Autodesk Fusion 360 part; units mm, degrees
(part 2 of 9)
sketch "Sketch3" plane through (0, 0, 5) normal (0, 0, 1) x (-1, 0, 0)
  line L0 (-9.15, 99.3) -> (-24.15, 99.3)
  line L1 (-24.15, 99.3) -> (-24.15, 114.3)
  line L2 (-24.15, 114.3) -> (-9.15, 114.3)
  line L3 (-9.15, 114.3) -> (-9.15, 99.3)
  line L4 (-42.475, 99.3) -> (-57.475, 99.3)
  line L5 (-57.475, 99.3) -> (-57.475, 114.3)
  line L6 (-57.475, 114.3) -> (-42.475, 114.3)
  line L7 (-42.475, 114.3) -> (-42.475, 99.3)
  line L8 (42.5, 114.3) -> (57.5, 114.3)
  line L9 (57.5, 114.3) -> (57.5, 99.3)
  line L10 (57.5, 99.3) -> (42.5, 99.3)
  line L11 (42.5, 99.3) -> (42.5, 114.3)
  line L12 (24.175, 99.3) -> (9.175, 99.3)
  line L13 (9.175, 99.3) -> (9.175, 114.3)
  line L14 (9.175, 114.3) -> (24.175, 114.3)
  line L15 (24.175, 114.3) -> (24.175, 99.3)
  line L16 (-76.5, 75.505) -> (-91.5, 75.505)
  line L17 (-91.5, 75.505) -> (-91.5, 90.505)
  line L18 (-91.5, 90.505) -> (-76.5, 90.505)
  line L19 (-76.5, 90.505) -> (-76.5, 75.505)
  line L20 (-59.7, 75.505) -> (-74.7, 75.505)
  line L21 (-74.7, 75.505) -> (-74.7, 90.505)
  line L22 (-74.7, 90.505) -> (-59.7, 90.505)
  line L23 (-59.7, 90.505) -> (-59.7, 75.505)
  line L24 (-42.9, 75.505) -> (-57.9, 75.505)
  line L25 (-57.9, 75.505) -> (-57.9, 90.505)
  line L26 (-57.9, 90.505) -> (-42.9, 90.505)
  line L27 (-42.9, 90.505) -> (-42.9, 75.505)
  line L28 (-9.3, -72.055) -> (-24.3, -72.055)
  line L29 (-24.3, -72.055) -> (-24.3, -57.055)
  line L30 (-24.3, -57.055) -> (-9.3, -57.055)
  line L31 (-9.3, -57.055) -> (-9.3, -72.055)
  line L32 (24.3, -72.055) -> (9.3, -72.055)
  line L33 (9.3, -72.055) -> (9.3, -57.055)
  line L34 (9.3, -57.055) -> (24.3, -57.055)
  line L35 (24.3, -57.055) -> (24.3, -72.055)
  line L36 (57.9, -72.055) -> (42.9, -72.055)
  line L37 (42.9, -72.055) -> (42.9, -57.055)
  line L38 (42.9, -57.055) -> (57.9, -57.055)
  line L39 (57.9, -57.055) -> (57.9, -72.055)
  line L40 (41.1, -72.055) -> (26.1, -72.055)
  line L41 (26.1, -72.055) -> (26.1, -57.055)
  line L42 (26.1, -57.055) -> (41.1, -57.055)
  line L43 (41.1, -57.055) -> (41.1, -72.055)
  line L44 (-76.5, -90.5) -> (-91.5, -90.5)
  line L45 (-91.5, -90.5) -> (-91.5, -75.5)
  line L46 (-91.5, -75.5) -> (-76.5, -75.5)
  line L47 (-76.5, -75.5) -> (-76.5, -90.5)
  line L48 (91.5, -72.055) -> (76.5, -72.055)
  line L49 (76.5, -72.055) -> (76.5, -57.055)
  line L50 (76.5, -57.055) -> (91.5, -57.055)
  line L51 (91.5, -57.055) -> (91.5, -72.055)
  line L52 (7.5, -72.055) -> (-7.5, -72.055)
  line L53 (-7.5, -72.055) -> (-7.5, -57.055)
  line L54 (-7.5, -57.055) -> (7.5, -57.055)
  line L55 (7.5, -57.055) -> (7.5, -72.055)
  line L56 (74.7, -72.055) -> (59.7, -72.055)
  line L57 (59.7, -72.055) -> (59.7, -57.055)
  line L58 (59.7, -57.055) -> (74.7, -57.055)
  line L59 (74.7, -57.055) -> (74.7, -72.055)
  line L60 (24.3, -90.5) -> (9.3, -90.5)
  line L61 (9.3, -90.5) -> (9.3, -75.5)
  line L62 (9.3, -75.5) -> (24.3, -75.5)
  line L63 (24.3, -75.5) -> (24.3, -90.5)
  line L64 (7.5, -90.5) -> (-7.5, -90.5)
  line L65 (-7.5, -90.5) -> (-7.5, -75.5)
  line L66 (-7.5, -75.5) -> (7.5, -75.5)
  line L67 (7.5, -75.5) -> (7.5, -90.5)
  line L68 (-59.7, -90.5) -> (-74.7, -90.5)
  line L69 (-74.7, -90.5) -> (-74.7, -75.5)
  line L70 (-74.7, -75.5) -> (-59.7, -75.5)
  line L71 (-59.7, -75.5) -> (-59.7, -90.5)
  line L72 (-9.3, -90.5) -> (-24.3, -90.5)
  line L73 (-24.3, -90.5) -> (-24.3, -75.5)
  line L74 (-24.3, -75.5) -> (-9.3, -75.5)
  line L75 (-9.3, -75.5) -> (-9.3, -90.5)
  line L76 (41.1, -90.5) -> (26.1, -90.5)
  line L77 (26.1, -90.5) -> (26.1, -75.5)
  line L78 (26.1, -75.5) -> (41.1, -75.5)
  line L79 (41.1, -75.5) -> (41.1, -90.5)
  line L80 (-26.1, -90.5) -> (-41.1, -90.5)
  line L81 (-41.1, -90.5) -> (-41.1, -75.5)
  line L82 (-41.1, -75.5) -> (-26.1, -75.5)
  line L83 (-26.1, -75.5) -> (-26.1, -90.5)
  line L84 (-42.9, -90.5) -> (-57.9, -90.5)
  line L85 (-57.9, -90.5) -> (-57.9, -75.5)
  line L86 (-57.9, -75.5) -> (-42.9, -75.5)
  line L87 (-42.9, -75.5) -> (-42.9, -90.5)
  circle A0 centre (110, 110) radius 1.6
  line L88 (76.5, -75.5) -> (91.5, -75.5)
  line L89 (91.5, -75.5) -> (91.5, -90.5)
  line L90 (91.5, -90.5) -> (76.5, -90.5)
  line L91 (76.5, -90.5) -> (76.5, -75.5)
  line L92 (74.7, -90.5) -> (59.7, -90.5)
  line L93 (59.7, -90.5) -> (59.7, -75.5)
  line L94 (59.7, -75.5) -> (74.7, -75.5)
  line L95 (74.7, -75.5) -> (74.7, -90.5)
  line L96 (57.9, -90.5) -> (42.9, -90.5)
  line L97 (42.9, -90.5) -> (42.9, -75.5)
  line L98 (42.9, -75.5) -> (57.9, -75.5)
  line L99 (57.9, -75.5) -> (57.9, -90.5)
  circle A1 centre (-110, -110) radius 1.6
  circle A2 centre (-110, 110) radius 1.6
  line L100 (-76.5, -72.055) -> (-91.5, -72.055)
  line L101 (-91.5, -72.055) -> (-91.5, -57.055)
  line L102 (-91.5, -57.055) -> (-76.5, -57.055)
  line L103 (-76.5, -57.055) -> (-76.5, -72.055)
  line L104 (91.5, -53.61) -> (76.5, -53.61)
  line L105 (76.5, -53.61) -> (76.5, -38.61)
  line L106 (76.5, -38.61) -> (91.5, -38.61)
  line L107 (91.5, -38.61) -> (91.5, -53.61)
  circle A3 centre (110, -110) radius 1.6
  line L108 (-42.9, -72.055) -> (-57.9, -72.055)
  line L109 (-57.9, -72.055) -> (-57.9, -57.055)
  line L110 (-57.9, -57.055) -> (-42.9, -57.055)
  line L111 (-42.9, -57.055) -> (-42.9, -72.055)
  line L112 (-26.1, -72.055) -> (-41.1, -72.055)
  line L113 (-41.1, -72.055) -> (-41.1, -57.055)
  line L114 (-41.1, -57.055) -> (-26.1, -57.055)
  line L115 (-26.1, -57.055) -> (-26.1, -72.055)
  line L116 (-59.7, -72.055) -> (-74.7, -72.055)
  line L117 (-74.7, -72.055) -> (-74.7, -57.055)
  line L118 (-74.7, -57.055) -> (-59.7, -57.055)
  line L119 (-59.7, -57.055) -> (-59.7, -72.055)
  line L120 (74.7, -53.61) -> (59.7, -53.61)
  line L121 (59.7, -53.61) -> (59.7, -38.61)
  line L122 (59.7, -38.61) -> (74.7, -38.61)
  line L123 (74.7, -38.61) -> (74.7, -53.61)
  line L124 (57.9, -53.61) -> (42.9, -53.61)
  line L125 (42.9, -53.61) -> (42.9, -38.61)
  line L126 (42.9, -38.61) -> (57.9, -38.61)
  line L127 (57.9, -38.61) -> (57.9, -53.61)
  line L128 (41.1, -35.165) -> (26.1, -35.165)
  line L129 (26.1, -35.165) -> (26.1, -20.165)
  line L130 (26.1, -20.165) -> (41.1, -20.165)
  line L131 (41.1, -20.165) -> (41.1, -35.165)
  line L132 (24.3, -35.165) -> (9.3, -35.165)
  line L133 (9.3, -35.165) -> (9.3, -20.165)
  line L134 (9.3, -20.165) -> (24.3, -20.165)
  line L135 (24.3, -20.165) -> (24.3, -35.165)
  line L136 (7.5, -35.165) -> (-7.5, -35.165)
  line L137 (-7.5, -35.165) -> (-7.5, -20.165)
  line L138 (-7.5, -20.165) -> (7.5, -20.165)
  line L139 (7.5, -20.165) -> (7.5, -35.165)
  line L140 (-26.1, -35.165) -> (-41.1, -35.165)
  line L141 (-41.1, -35.165) -> (-41.1, -20.165)
  line L142 (-41.1, -20.165) -> (-26.1, -20.165)
  line L143 (-26.1, -20.165) -> (-26.1, -35.165)
  line L144 (-9.3, -35.165) -> (-24.3, -35.165)
  line L145 (-24.3, -35.165) -> (-24.3, -20.165)
  line L146 (-24.3, -20.165) -> (-9.3, -20.165)
  line L147 (-9.3, -20.165) -> (-9.3, -35.165)
  line L148 (-42.9, -35.165) -> (-57.9, -35.165)
  line L149 (-57.9, -35.165) -> (-57.9, -20.165)
  line L150 (-57.9, -20.165) -> (-42.9, -20.165)
  line L151 (-42.9, -20.165) -> (-42.9, -35.165)
  line L152 (-59.7, -35.165) -> (-74.7, -35.165)
  line L153 (-74.7, -35.165) -> (-74.7, -20.165)
  line L154 (-74.7, -20.165) -> (-59.7, -20.165)
  line L155 (-59.7, -20.165) -> (-59.7, -35.165)
  line L156 (41.1, -16.72) -> (26.1, -16.72)
  line L157 (26.1, -16.72) -> (26.1, -1.72)
  line L158 (26.1, -1.72) -> (41.1, -1.72)
  line L159 (41.1, -1.72) -> (41.1, -16.72)
  line L160 (91.5, -16.72) -> (76.5, -16.72)
  line L161 (76.5, -16.72) -> (76.5, -1.72)
  line L162 (76.5, -1.72) -> (91.5, -1.72)
  line L163 (91.5, -1.72) -> (91.5, -16.72)
  line L164 (74.7, -16.72) -> (59.7, -16.72)
  line L165 (59.7, -16.72) -> (59.7, -1.72)
  line L166 (59.7, -1.72) -> (74.7, -1.72)
  line L167 (74.7, -1.72) -> (74.7, -16.72)
  line L168 (57.9, -16.72) -> (42.9, -16.72)
  line L169 (42.9, -16.72) -> (42.9, -1.72)
  line L170 (42.9, -1.72) -> (57.9, -1.72)
  line L171 (57.9, -1.72) -> (57.9, -16.72)
  line L172 (24.3, -16.72) -> (9.3, -16.72)
  line L173 (9.3, -16.72) -> (9.3, -1.72)
  line L174 (9.3, -1.72) -> (24.3, -1.72)
  line L175 (24.3, -1.72) -> (24.3, -16.72)
  line L176 (7.5, -16.72) -> (-7.5, -16.72)
  line L177 (-7.5, -16.72) -> (-7.5, -1.72)
  line L178 (-7.5, -1.72) -> (7.5, -1.72)
  line L179 (7.5, -1.72) -> (7.5, -16.72)
  line L180 (-76.5, -35.165) -> (-91.5, -35.165)
  line L181 (-91.5, -35.165) -> (-91.5, -20.165)
  line L182 (-91.5, -20.165) -> (-76.5, -20.165)
  line L183 (-76.5, -20.165) -> (-76.5, -35.165)
  line L184 (-42.9, -16.72) -> (-57.9, -16.72)
  line L185 (-57.9, -16.72) -> (-57.9, -1.72)
  line L186 (-57.9, -1.72) -> (-42.9, -1.72)
  line L187 (-42.9, -1.72) -> (-42.9, -16.72)
  line L188 (-59.7, -16.72) -> (-74.7, -16.72)
  line L189 (-74.7, -16.72) -> (-74.7, -1.72)
  line L190 (-74.7, -1.72) -> (-59.7, -1.72)
  line L191 (-59.7, -1.72) -> (-59.7, -16.72)
  line L192 (-9.3, -16.72) -> (-24.3, -16.72)
  line L193 (-24.3, -16.72) -> (-24.3, -1.72)
  line L194 (-24.3, -1.72) -> (-9.3, -1.72)
  line L195 (-9.3, -1.72) -> (-9.3, -16.72)
  line L196 (-26.1, -16.72) -> (-41.1, -16.72)
  line L197 (-41.1, -16.72) -> (-41.1, -1.72)
  line L198 (-41.1, -1.72) -> (-26.1, -1.72)
  line L199 (-26.1, -1.72) -> (-26.1, -16.72)
  line L200 (-9.3, -53.61) -> (-24.3, -53.61)
  line L201 (-24.3, -53.61) -> (-24.3, -38.61)
  line L202 (-24.3, -38.61) -> (-9.3, -38.61)
  line L203 (-9.3, -38.61) -> (-9.3, -53.61)
  line L204 (7.5, -53.61) -> (-7.5, -53.61)
  line L205 (-7.5, -53.61) -> (-7.5, -38.61)
  line L206 (-7.5, -38.61) -> (7.5, -38.61)
  line L207 (7.5, -38.61) -> (7.5, -53.61)
  line L208 (24.3, -53.61) -> (9.3, -53.61)
  line L209 (9.3, -53.61) -> (9.3, -38.61)
  line L210 (9.3, -38.61) -> (24.3, -38.61)
  line L211 (24.3, -38.61) -> (24.3, -53.61)
  line L212 (41.1, -53.61) -> (26.1, -53.61)
  line L213 (26.1, -53.61) -> (26.1, -38.61)
  line L214 (26.1, -38.61) -> (41.1, -38.61)
  line L215 (41.1, -38.61) -> (41.1, -53.61)
  line L216 (91.5, -35.165) -> (76.5, -35.165)
  line L217 (76.5, -35.165) -> (76.5, -20.165)
  line L218 (76.5, -20.165) -> (91.5, -20.165)
  line L219 (91.5, -20.165) -> (91.5, -35.165)
  line L220 (57.9, -35.165) -> (42.9, -35.165)
  line L221 (42.9, -35.165) -> (42.9, -20.165)
  line L222 (42.9, -20.165) -> (57.9, -20.165)
  line L223 (57.9, -20.165) -> (57.9, -35.165)
  line L224 (-76.5, -53.61) -> (-91.5, -53.61)
  line L225 (-91.5, -53.61) -> (-91.5, -38.61)
  line L226 (-91.5, -38.61) -> (-76.5, -38.61)
  line L227 (-76.5, -38.61) -> (-76.5, -53.61)
  line L228 (-59.7, -53.61) -> (-74.7, -53.61)
  line L229 (-74.7, -53.61) -> (-74.7, -38.61)
  line L230 (-74.7, -38.61) -> (-59.7, -38.61)
  line L231 (-59.7, -38.61) -> (-59.7, -53.61)
  line L232 (-26.1, -53.61) -> (-41.1, -53.61)
  line L233 (-41.1, -53.61) -> (-41.1, -38.61)
  line L234 (-41.1, -38.61) -> (-26.1, -38.61)
  line L235 (-26.1, -38.61) -> (-26.1, -53.61)
  line L236 (74.7, -35.165) -> (59.7, -35.165)
  line L237 (59.7, -35.165) -> (59.7, -20.165)
  line L238 (59.7, -20.165) -> (74.7, -20.165)
  line L239 (74.7, -20.165) -> (74.7, -35.165)
  line L240 (-42.9, -53.61) -> (-57.9, -53.61)
  line L241 (-57.9, -53.61) -> (-57.9, -38.61)
  line L242 (-57.9, -38.61) -> (-42.9, -38.61)
  line L243 (-42.9, -38.61) -> (-42.9, -53.61)
  line L244 (41.1, 38.615) -> (26.1, 38.615)
  line L245 (26.1, 38.615) -> (26.1, 53.615)
  line L246 (26.1, 53.615) -> (41.1, 53.615)
  line L247 (41.1, 53.615) -> (41.1, 38.615)
  line L248 (91.5, 38.615) -> (76.5, 38.615)
  line L249 (76.5, 38.615) -> (76.5, 53.615)
  line L250 (76.5, 53.615) -> (91.5, 53.615)
  line L251 (91.5, 53.615) -> (91.5, 38.615)
  line L252 (7.5, 38.615) -> (-7.5, 38.615)
  line L253 (-7.5, 38.615) -> (-7.5, 53.615)
  line L254 (-7.5, 53.615) -> (7.5, 53.615)
  line L255 (7.5, 53.615) -> (7.5, 38.615)
  line L256 (74.7, 38.615) -> (59.7, 38.615)
  line L257 (59.7, 38.615) -> (59.7, 53.615)
  line L258 (59.7, 53.615) -> (74.7, 53.615)
  line L259 (74.7, 53.615) -> (74.7, 38.615)
  line L260 (24.3, 38.615) -> (9.3, 38.615)
  line L261 (9.3, 38.615) -> (9.3, 53.615)
  line L262 (9.3, 53.615) -> (24.3, 53.615)
  line L263 (24.3, 53.615) -> (24.3, 38.615)
  line L264 (57.9, 38.615) -> (42.9, 38.615)
  line L265 (42.9, 38.615) -> (42.9, 53.615)
  line L266 (42.9, 53.615) -> (57.9, 53.615)
  line L267 (57.9, 53.615) -> (57.9, 38.615)
  line L268 (91.5, 57.06) -> (76.5, 57.06)
  line L269 (76.5, 57.06) -> (76.5, 72.06)
  line L270 (76.5, 72.06) -> (91.5, 72.06)
  line L271 (91.5, 72.06) -> (91.5, 57.06)
  line L272 (-59.7, 38.615) -> (-74.7, 38.615)
  line L273 (-74.7, 38.615) -> (-74.7, 53.615)
  line L274 (-74.7, 53.615) -> (-59.7, 53.615)
  line L275 (-59.7, 53.615) -> (-59.7, 38.615)
  line L276 (-42.9, 38.615) -> (-57.9, 38.615)
  line L277 (-57.9, 38.615) -> (-57.9, 53.615)
  line L278 (-57.9, 53.615) -> (-42.9, 53.615)
  line L279 (-42.9, 53.615) -> (-42.9, 38.615)
  line L280 (-26.1, 38.615) -> (-41.1, 38.615)
  line L281 (-41.1, 38.615) -> (-41.1, 53.615)
  line L282 (-41.1, 53.615) -> (-26.1, 53.615)
  line L283 (-26.1, 53.615) -> (-26.1, 38.615)
  line L284 (-76.5, 38.615) -> (-91.5, 38.615)
  line L285 (-91.5, 38.615) -> (-91.5, 53.615)
  line L286 (-91.5, 53.615) -> (-76.5, 53.615)
  line L287 (-76.5, 53.615) -> (-76.5, 38.615)
  line L288 (-9.3, 38.615) -> (-24.3, 38.615)
  line L289 (-24.3, 38.615) -> (-24.3, 53.615)
  line L290 (-24.3, 53.615) -> (-9.3, 53.615)
  line L291 (-9.3, 53.615) -> (-9.3, 38.615)
  line L292 (57.9, 57.06) -> (42.9, 57.06)
  line L293 (42.9, 57.06) -> (42.9, 72.06)
  line L294 (42.9, 72.06) -> (57.9, 72.06)
  line L295 (57.9, 72.06) -> (57.9, 57.06)
  line L296 (24.3, 57.06) -> (9.3, 57.06)
  line L297 (9.3, 57.06) -> (9.3, 72.06)
  line L298 (9.3, 72.06) -> (24.3, 72.06)
  line L299 (24.3, 72.06) -> (24.3, 57.06)
  line L300 (41.1, 57.06) -> (26.1, 57.06)
  line L301 (26.1, 57.06) -> (26.1, 72.06)
  line L302 (26.1, 72.06) -> (41.1, 72.06)
  line L303 (41.1, 72.06) -> (41.1, 57.06)
  line L304 (-9.3, 57.06) -> (-24.3, 57.06)
  line L305 (-24.3, 57.06) -> (-24.3, 72.06)
  line L306 (-24.3, 72.06) -> (-9.3, 72.06)
  line L307 (-9.3, 72.06) -> (-9.3, 57.06)
  line L308 (7.5, 57.06) -> (-7.5, 57.06)
  line L309 (-7.5, 57.06) -> (-7.5, 72.06)
  line L310 (-7.5, 72.06) -> (7.5, 72.06)
  line L311 (7.5, 72.06) -> (7.5, 57.06)
  line L312 (74.7, 57.06) -> (59.7, 57.06)
  line L313 (59.7, 57.06) -> (59.7, 72.06)
  line L314 (59.7, 72.06) -> (74.7, 72.06)
  line L315 (74.7, 72.06) -> (74.7, 57.06)
  line L316 (-26.1, 57.06) -> (-41.1, 57.06)
  line L317 (-41.1, 57.06) -> (-41.1, 72.06)
  line L318 (-41.1, 72.06) -> (-26.1, 72.06)
  line L319 (-26.1, 72.06) -> (-26.1, 57.06)
  line L320 (-42.9, 57.06) -> (-57.9, 57.06)
  line L321 (-57.9, 57.06) -> (-57.9, 72.06)
  line L322 (-57.9, 72.06) -> (-42.9, 72.06)
  line L323 (-42.9, 72.06) -> (-42.9, 57.06)
  line L324 (57.9, 1.725) -> (42.9, 1.725)
  line L325 (42.9, 1.725) -> (42.9, 16.725)
  line L326 (42.9, 16.725) -> (57.9, 16.725)
  line L327 (57.9, 16.725) -> (57.9, 1.725)
  line L328 (41.1, 1.725) -> (26.1, 1.725)
  line L329 (26.1, 1.725) -> (26.1, 16.725)
  line L330 (26.1, 16.725) -> (41.1, 16.725)
  line L331 (41.1, 16.725) -> (41.1, 1.725)
  line L332 (91.5, 1.725) -> (76.5, 1.725)
  line L333 (76.5, 1.725) -> (76.5, 16.725)
  line L334 (76.5, 16.725) -> (91.5, 16.725)
  line L335 (91.5, 16.725) -> (91.5, 1.725)
  line L336 (-76.5, -16.72) -> (-91.5, -16.72)
  line L337 (-91.5, -16.72) -> (-91.5, -1.72)
  line L338 (-91.5, -1.72) -> (-76.5, -1.72)
  line L339 (-76.5, -1.72) -> (-76.5, -16.72)
  line L340 (74.7, 1.725) -> (59.7, 1.725)
  line L341 (59.7, 1.725) -> (59.7, 16.725)
  line L342 (59.7, 16.725) -> (74.7, 16.725)
  line L343 (74.7, 16.725) -> (74.7, 1.725)
  line L344 (-9.3, 1.725) -> (-24.3, 1.725)
  line L345 (-24.3, 1.725) -> (-24.3, 16.725)
  line L346 (-24.3, 16.725) -> (-9.3, 16.725)
  line L347 (-9.3, 16.725) -> (-9.3, 1.725)
  line L348 (-26.1, 1.725) -> (-41.1, 1.725)
  line L349 (-41.1, 1.725) -> (-41.1, 16.725)
  line L350 (-41.1, 16.725) -> (-26.1, 16.725)
  line L351 (-26.1, 16.725) -> (-26.1, 1.725)
  line L352 (24.3, 1.725) -> (9.3, 1.725)
  line L353 (9.3, 1.725) -> (9.3, 16.725)
  line L354 (9.3, 16.725) -> (24.3, 16.725)
  line L355 (24.3, 16.725) -> (24.3, 1.725)
  line L356 (-42.9, 1.725) -> (-57.9, 1.725)
  line L357 (-57.9, 1.725) -> (-57.9, 16.725)
  line L358 (-57.9, 16.725) -> (-42.9, 16.725)
  line L359 (-42.9, 16.725) -> (-42.9, 1.725)
  line L360 (7.5, 1.725) -> (-7.5, 1.725)
  line L361 (-7.5, 1.725) -> (-7.5, 16.725)
  line L362 (-7.5, 16.725) -> (7.5, 16.725)
  line L363 (7.5, 16.725) -> (7.5, 1.725)
  line L364 (-59.7, 1.725) -> (-74.7, 1.725)
  line L365 (-74.7, 1.725) -> (-74.7, 16.725)
  line L366 (-74.7, 16.725) -> (-59.7, 16.725)
  line L367 (-59.7, 16.725) -> (-59.7, 1.725)
  line L368 (74.7, 20.17) -> (59.7, 20.17)
  line L369 (59.7, 20.17) -> (59.7, 35.17)
  line L370 (59.7, 35.17) -> (74.7, 35.17)
  line L371 (74.7, 35.17) -> (74.7, 20.17)
  line L372 (57.9, 20.17) -> (42.9, 20.17)
  line L373 (42.9, 20.17) -> (42.9, 35.17)
  line L374 (42.9, 35.17) -> (57.9, 35.17)
  line L375 (57.9, 35.17) -> (57.9, 20.17)
  line L376 (-76.5, 1.725) -> (-91.5, 1.725)
  line L377 (-91.5, 1.725) -> (-91.5, 16.725)
  line L378 (-91.5, 16.725) -> (-76.5, 16.725)
  line L379 (-76.5, 16.725) -> (-76.5, 1.725)
  line L380 (7.5, 20.17) -> (-7.5, 20.17)
  line L381 (-7.5, 20.17) -> (-7.5, 35.17)
  line L382 (-7.5, 35.17) -> (7.5, 35.17)
  line L383 (7.5, 35.17) -> (7.5, 20.17)
  line L384 (24.3, 20.17) -> (9.3, 20.17)
  line L385 (9.3, 20.17) -> (9.3, 35.17)
  line L386 (9.3, 35.17) -> (24.3, 35.17)
  line L387 (24.3, 35.17) -> (24.3, 20.17)
  line L388 (91.5, 20.17) -> (76.5, 20.17)
  line L389 (76.5, 20.17) -> (76.5, 35.17)
  line L390 (76.5, 35.17) -> (91.5, 35.17)
  line L391 (91.5, 35.17) -> (91.5, 20.17)
  line L392 (41.1, 20.17) -> (26.1, 20.17)
  line L393 (26.1, 20.17) -> (26.1, 35.17)
  line L394 (26.1, 35.17) -> (41.1, 35.17)
  line L395 (41.1, 35.17) -> (41.1, 20.17)
  line L396 (-59.7, 20.17) -> (-74.7, 20.17)
  line L397 (-74.7, 20.17) -> (-74.7, 35.17)
  line L398 (-74.7, 35.17) -> (-59.7, 35.17)
  line L399 (-59.7, 35.17) -> (-59.7, 20.17)
  line L400 (-9.3, 20.17) -> (-24.3, 20.17)
  line L401 (-24.3, 20.17) -> (-24.3, 35.17)
  line L402 (-24.3, 35.17) -> (-9.3, 35.17)
  line L403 (-9.3, 35.17) -> (-9.3, 20.17)
  line L404 (-26.1, 20.17) -> (-41.1, 20.17)
  line L405 (-41.1, 20.17) -> (-41.1, 35.17)
  line L406 (-41.1, 35.17) -> (-26.1, 35.17)
  line L407 (-26.1, 35.17) -> (-26.1, 20.17)
  line L408 (-42.9, 20.17) -> (-57.9, 20.17)
  line L409 (-57.9, 20.17) -> (-57.9, 35.17)
  line L410 (-57.9, 35.17) -> (-42.9, 35.17)
  line L411 (-42.9, 35.17) -> (-42.9, 20.17)
  line L412 (-76.5, 20.17) -> (-91.5, 20.17)
  line L413 (-91.5, 20.17) -> (-91.5, 35.17)
  line L414 (-91.5, 35.17) -> (-76.5, 35.17)
  line L415 (-76.5, 35.17) -> (-76.5, 20.17)
  line L416 (-76.5, 57.06) -> (-91.5, 57.06)
  line L417 (-91.5, 57.06) -> (-91.5, 72.06)
  line L418 (-91.5, 72.06) -> (-76.5, 72.06)
  line L419 (-76.5, 72.06) -> (-76.5, 57.06)
  line L420 (57.9, 75.505) -> (42.9, 75.505)
  line L421 (42.9, 75.505) -> (42.9, 90.505)
  line L422 (42.9, 90.505) -> (57.9, 90.505)
  line L423 (57.9, 90.505) -> (57.9, 75.505)
  line L424 (-59.7, 57.06) -> (-74.7, 57.06)
  line L425 (-74.7, 57.06) -> (-74.7, 72.06)
  line L426 (-74.7, 72.06) -> (-59.7, 72.06)
  line L427 (-59.7, 72.06) -> (-59.7, 57.06)
  line L428 (91.5, 75.505) -> (76.5, 75.505)
  line L429 (76.5, 75.505) -> (76.5, 90.505)
  line L430 (76.5, 90.505) -> (91.5, 90.505)
  line L431 (91.5, 90.505) -> (91.5, 75.505)
  line L432 (74.7, 75.505) -> (59.7, 75.505)
  line L433 (59.7, 75.505) -> (59.7, 90.505)
  line L434 (59.7, 90.505) -> (74.7, 90.505)
  line L435 (74.7, 90.505) -> (74.7, 75.505)
  line L436 (7.5, 75.505) -> (-7.5, 75.505)
  line L437 (-7.5, 75.505) -> (-7.5, 90.505)
  line L438 (-7.5, 90.505) -> (7.5, 90.505)
  line L439 (7.5, 90.505) -> (7.5, 75.505)
  line L440 (-9.3, 75.505) -> (-24.3, 75.505)
  line L441 (-24.3, 75.505) -> (-24.3, 90.505)
  line L442 (-24.3, 90.505) -> (-9.3, 90.505)
  line L443 (-9.3, 90.505) -> (-9.3, 75.505)
  line L444 (24.3, 75.505) -> (9.3, 75.505)
  line L445 (9.3, 75.505) -> (9.3, 90.505)
  line L446 (9.3, 90.505) -> (24.3, 90.505)
  line L447 (24.3, 90.505) -> (24.3, 75.505)
  line L448 (41.1, 75.505) -> (26.1, 75.505)
  line L449 (26.1, 75.505) -> (26.1, 90.505)
  line L450 (26.1, 90.505) -> (41.1, 90.505)
  line L451 (41.1, 90.505) -> (41.1, 75.505)
  line L452 (-26.1, 75.505) -> (-41.1, 75.505)
  line L453 (-41.1, 75.505) -> (-41.1, 90.505)
  line L454 (-41.1, 90.505) -> (-26.1, 90.505)
  line L455 (-26.1, 90.505) -> (-26.1, 75.505)
  line L456 (-117.5, 117.5) -> (-117.5, -117.5)
  line L457 (-117.5, -117.5) -> (117.5, -117.5)
  line L458 (117.5, -117.5) -> (117.5, 117.5)
  line L459 (117.5, 117.5) -> (-117.5, 117.5)
  line L460 (-5.65, 109) -> (-10.65, 109)
  line L461 (-10.65, 109) -> (-10.65, 116)
  line L462 (-10.65, 116) -> (-5.65, 116)
  line L463 (-5.65, 116) -> (-5.65, 109)
  dimension "d36" = 3.5
  dimension "d37" = 8.5
  dimension "d38" = 7
  dimension "d39" = 5
  constraint horizontal L460
  constraint vertical L461
  constraint horizontal L462
  constraint vertical L463
  measures "d36" distance of L3 L463
  measures "d37" distance of L459 L460
  measures "d38" distance of L460 L462
  measures "d39" distance of L461 L463
extrude "Extrude2" cut sketch "Sketch3" along normal blind -7 and the other way blind 4 contours L2 L3 L460 L461 L462 L463
sketch "Sketch5" plane through (0, 0, 0) normal (0, 0, 1) x (1, 0, 0)
  line L0 (-150, 150) -> (150, 150)
  line L1 (150, 150) -> (150, -150)
  line L2 (150, -150) -> (-150, -150)
  line L3 (-150, -150) -> (-150, 150)
  spline S0 degree 3 poles (102.2213, -100.0075) (102.2213, -101.2499) (101.2142, -102.2576) (99.9715, -102.2576) knots 0 0 0 0 1 1 1 1
  spline S1 degree 3 poles (99.9715, -102.2576) (98.7292, -102.2576) (97.7218, -101.2502) (97.7218, -100.0075) knots 0 0 0 0 1 1 1 1
  spline S2 degree 3 poles (97.7218, -100.0075) (97.7218, -98.7648) (98.7292, -97.7574) (99.9715, -97.7574) knots 0 0 0 0 1 1 1 1
  spline S3 degree 3 poles (99.9715, -97.7574) (101.2142, -97.7577) (102.2213, -98.7652) (102.2213, -100.0075) knots 0 0 0 0 1 1 1 1
  circle A0 centre (99.9716, -100.0075) radius 2.2497
  spline S4 degree 3 poles (-97.7546, -100.0075) (-97.7546, -101.2499) (-98.7617, -102.2576) (-100.0043, -102.2576) knots 0 0 0 0 1 1 1 1
  spline S5 degree 3 poles (-100.0043, -102.2576) (-101.2467, -102.2576) (-102.2541, -101.2502) (-102.2541, -100.0075) knots 0 0 0 0 1 1 1 1
  spline S6 degree 3 poles (-102.2541, -100.0075) (-102.2541, -98.7648) (-101.2467, -97.7574) (-100.0043, -97.7574) knots 0 0 0 0 1 1 1 1
  spline S7 degree 3 poles (-100.0043, -97.7574) (-98.7617, -97.7577) (-97.7546, -98.7652) (-97.7546, -100.0075) knots 0 0 0 0 1 1 1 1
  circle A1 centre (-100.0044, -100.0075) radius 2.2497
  spline S8 degree 3 poles (-97.7546, 99.9677) (-97.7546, 98.7254) (-98.7617, 97.7179) (-100.0043, 97.7179) knots 0 0 0 0 1 1 1 1
  spline S9 degree 3 poles (-100.0043, 97.7179) (-101.2467, 97.7179) (-102.2541, 98.7254) (-102.2541, 99.9677) knots 0 0 0 0 1 1 1 1
  spline S10 degree 3 poles (-102.2541, 99.9677) (-102.2541, 101.21) (-101.2467, 102.2175) (-100.0043, 102.2175) knots 0 0 0 0 1 1 1 1
  spline S11 degree 3 poles (-100.0043, 102.2175) (-98.7617, 102.2175) (-97.7546, 101.21) (-97.7546, 99.9677) knots 0 0 0 0 1 1 1 1
  circle A2 centre (-100.0044, 99.9677) radius 2.2497
  spline S12 degree 3 poles (102.2213, 99.9677) (102.2213, 98.7254) (101.2142, 97.7179) (99.9715, 97.7179) knots 0 0 0 0 1 1 1 1
  spline S13 degree 3 poles (99.9715, 97.7179) (98.7292, 97.7179) (97.7218, 98.7254) (97.7218, 99.9677) knots 0 0 0 0 1 1 1 1
  spline S14 degree 3 poles (97.7218, 99.9677) (97.7218, 101.21) (98.7292, 102.2175) (99.9715, 102.2175) knots 0 0 0 0 1 1 1 1
  spline S15 degree 3 poles (99.9715, 102.2175) (101.2142, 102.2175) (102.2213, 101.21) (102.2213, 99.9677) knots 0 0 0 0 1 1 1 1
  circle A3 centre (99.9716, 99.9677) radius 2.2497
  line L4 (-87.1879, 79.2853) -> (-81.5345, 79.2853) construction
  line L5 (-81.5345, 79.2853) -> (-81.5345, 89.8687) construction
  line L6 (-81.5345, 89.8687) -> (-87.1879, 89.8687) construction
  line L7 (-87.1879, 89.8687) -> (-87.1879, 79.2853) construction
  line L8 (-70.5192, 79.2853) -> (-64.4885, 79.2853) construction
  line L9 (-64.4885, 79.2853) -> (-64.4885, 89.8687) construction
  line L10 (-64.4885, 89.8687) -> (-70.5192, 89.8687) construction
  line L11 (-70.5192, 89.8687) -> (-70.5192, 79.2853) construction
  line L12 (-53.8504, 79.2853) -> (-47.5872, 79.2853) construction
  line L13 (-47.5872, 79.2853) -> (-47.5872, 89.8687) construction
  line L14 (-47.5872, 89.8687) -> (-53.8504, 89.8687) construction
  line L15 (-53.8504, 89.8687) -> (-53.8504, 79.2853) construction
  line L16 (-33.6817, 79.2853) -> (-32.6791, 79.2853) construction
  line L17 (-32.6791, 79.2853) -> (-32.6791, 89.8687) construction
  line L18 (-32.6791, 89.8687) -> (-33.6817, 89.8687) construction
  line L19 (-33.6817, 89.8687) -> (-33.6817, 79.2853) construction
  line L20 (-20.5129, 79.2853) -> (-14.4823, 79.2853) construction
  line L21 (-14.4823, 79.2853) -> (-14.4823, 89.8687) construction
  line L22 (-14.4823, 89.8687) -> (-20.5129, 89.8687) construction
  line L23 (-20.5129, 89.8687) -> (-20.5129, 79.2853) construction
  line L24 (-3.8442, 79.2853) -> (2.1606, 79.2853) construction
  line L25 (2.1606, 79.2853) -> (2.1606, 89.8687) construction
  line L26 (2.1606, 89.8687) -> (-3.8442, 89.8687) construction
  line L27 (-3.8442, 89.8687) -> (-3.8442, 79.2853) construction
  line L28 (12.8246, 79.2853) -> (17.5581, 79.2853) construction
  line L29 (17.5581, 79.2853) -> (17.5581, 89.8687) construction
  line L30 (17.5581, 89.8687) -> (12.8246, 89.8687) construction
  line L31 (12.8246, 89.8687) -> (12.8246, 79.2853) construction
  line L32 (29.4933, 79.2853) -> (34.6041, 79.2853) construction
  line L33 (34.6041, 79.2853) -> (34.6041, 89.8687) construction
  line L34 (34.6041, 89.8687) -> (29.4933, 89.8687) construction
  line L35 (29.4933, 89.8687) -> (29.4933, 79.2853) construction
  line L36 (46.1621, 79.2853) -> (52.1204, 79.2853) construction
  line L37 (52.1204, 79.2853) -> (52.1204, 89.8687) construction
  line L38 (52.1204, 89.8687) -> (46.1621, 89.8687) construction
  line L39 (46.1621, 89.8687) -> (46.1621, 79.2853) construction
  line L40 (62.8308, 79.2853) -> (68.7995, 79.2853) construction
  line L41 (68.7995, 79.2853) -> (68.7995, 89.8687) construction
  line L42 (68.7995, 89.8687) -> (62.8308, 89.8687) construction
  line L43 (62.8308, 89.8687) -> (62.8308, 79.2853) construction
  line L44 (79.4996, 79.2853) -> (84.6104, 79.2853) construction
  line L45 (84.6104, 79.2853) -> (84.6104, 89.8687) construction
  line L46 (84.6104, 89.8687) -> (79.4996, 89.8687) construction
  line L47 (79.4996, 89.8687) -> (79.4996, 79.2853) construction
  line L48 (96.1683, 79.2853) -> (102.5183, 79.2853) construction
  line L49 (102.5183, 79.2853) -> (102.5183, 89.8687) construction
  line L50 (102.5183, 89.8687) -> (96.1683, 89.8687) construction
  line L51 (96.1683, 89.8687) -> (96.1683, 79.2853) construction
  line L52 (-87.1879, 60.7853) -> (-81.1986, 60.7853) construction
  line L53 (-81.1986, 60.7853) -> (-81.1986, 71.3687) construction
  line L54 (-81.1986, 71.3687) -> (-87.1879, 71.3687) construction
  line L55 (-87.1879, 71.3687) -> (-87.1879, 60.7853) construction
  line L56 (-70.5192, 60.7853) -> (-64.8658, 60.7853) construction
  line L57 (-64.8658, 60.7853) -> (-64.8658, 71.3687) construction
  line L58 (-64.8658, 71.3687) -> (-70.5192, 71.3687) construction
  line L59 (-70.5192, 71.3687) -> (-70.5192, 60.7853) construction
  line L60 (-53.8504, 60.7853) -> (-47.9076, 60.7853) construction
  line L61 (-47.9076, 60.7853) -> (-47.9076, 71.3687) construction
  line L62 (-47.9076, 71.3687) -> (-53.8504, 71.3687) construction
  line L63 (-53.8504, 71.3687) -> (-53.8504, 60.7853) construction
  line L64 (-37.1817, 60.7853) -> (-31.213, 60.7853) construction
  line L65 (-31.213, 60.7853) -> (-31.213, 71.3687) construction
  line L66 (-31.213, 71.3687) -> (-37.1817, 71.3687) construction
  line L67 (-37.1817, 71.3687) -> (-37.1817, 60.7853) construction
  line L68 (-20.5129, 60.7853) -> (-14.5236, 60.7853) construction
  line L69 (-14.5236, 60.7853) -> (-14.5236, 71.3687) construction
  line L70 (-14.5236, 71.3687) -> (-20.5129, 71.3687) construction
  line L71 (-20.5129, 71.3687) -> (-20.5129, 60.7853) construction
  line L72 (-3.8442, 60.7853) -> (5.8968, 60.7853) construction
  line L73 (5.8968, 60.7853) -> (5.8968, 71.3687) construction
  line L74 (5.8968, 71.3687) -> (-3.8442, 71.3687) construction
  line L75 (-3.8442, 71.3687) -> (-3.8442, 60.7853) construction
  line L76 (12.8246, 60.7853) -> (19.9146, 60.7853) construction
  line L77 (19.9146, 60.7853) -> (19.9146, 71.3687) construction
  line L78 (19.9146, 71.3687) -> (12.8246, 71.3687) construction
  line L79 (12.8246, 71.3687) -> (12.8246, 60.7853) construction
  line L80 (29.4933, 60.7853) -> (35.462, 60.7853) construction
  line L81 (35.462, 60.7853) -> (35.462, 71.3687) construction
  line L82 (35.462, 71.3687) -> (29.4933, 71.3687) construction
  line L83 (29.4933, 71.3687) -> (29.4933, 60.7853) construction
  line L84 (46.1621, 60.7853) -> (52.1514, 60.7853) construction
  line L85 (52.1514, 60.7853) -> (52.1514, 71.3687) construction
  line L86 (52.1514, 71.3687) -> (46.1621, 71.3687) construction
  line L87 (46.1621, 71.3687) -> (46.1621, 60.7853) construction
  line L88 (66.3308, 60.7853) -> (67.3334, 60.7853) construction
  line L89 (67.3334, 60.7853) -> (67.3334, 71.3687) construction
  line L90 (67.3334, 71.3687) -> (66.3308, 71.3687) construction
  line L91 (66.3308, 71.3687) -> (66.3308, 60.7853) construction
  line L92 (79.4996, 60.7853) -> (86.5069, 60.7853) construction
  line L93 (86.5069, 60.7853) -> (86.5069, 71.3687) construction
  line L94 (86.5069, 71.3687) -> (79.4996, 71.3687) construction
  line L95 (79.4996, 71.3687) -> (79.4996, 60.7853) construction
  line L96 (96.1683, 60.7853) -> (102.5183, 60.7853) construction
  line L97 (102.5183, 60.7853) -> (102.5183, 71.3687) construction
  line L98 (102.5183, 71.3687) -> (96.1683, 71.3687) construction
  line L99 (96.1683, 71.3687) -> (96.1683, 60.7853) construction
  line L100 (-87.1879, 42.2853) -> (-80.9247, 42.2853) construction
  line L101 (-80.9247, 42.2853) -> (-80.9247, 52.8686) construction
  line L102 (-80.9247, 52.8686) -> (-87.1879, 52.8686) construction
  line L103 (-87.1879, 52.8686) -> (-87.1879, 42.2853) construction
  line L104 (-70.5192, 42.2853) -> (-63.8426, 42.2853) construction
  line L105 (-63.8426, 42.2853) -> (-63.8426, 52.8686) construction
  line L106 (-63.8426, 52.8686) -> (-70.5192, 52.8686) construction
  line L107 (-70.5192, 52.8686) -> (-70.5192, 42.2853) construction
  line L108 (-53.8504, 42.2853) -> (-48.197, 42.2853) construction
  line L109 (-48.197, 42.2853) -> (-48.197, 52.8686) construction
  line L110 (-48.197, 52.8686) -> (-53.8504, 52.8686) construction
  line L111 (-53.8504, 52.8686) -> (-53.8504, 42.2853) construction
  line L112 (-33.6817, 42.2853) -> (-32.6791, 42.2853) construction
  line L113 (-32.6791, 42.2853) -> (-32.6791, 52.8686) construction
  line L114 (-32.6791, 52.8686) -> (-33.6817, 52.8686) construction
  line L115 (-33.6817, 52.8686) -> (-33.6817, 42.2853) construction
  line L116 (-20.5129, 42.2853) -> (-13.5831, 42.2853) construction
  line L117 (-13.5831, 42.2853) -> (-13.5831, 52.8686) construction
  line L118 (-13.5831, 52.8686) -> (-20.5129, 52.8686) construction
  line L119 (-20.5129, 52.8686) -> (-20.5129, 42.2853) construction
  line L120 (-0.3442, 42.2853) -> (0.6584, 42.2853) construction
  line L121 (0.6584, 42.2853) -> (0.6584, 52.8686) construction
  line L122 (0.6584, 52.8686) -> (-0.3442, 52.8686) construction
  line L123 (-0.3442, 52.8686) -> (-0.3442, 42.2853) construction
  line L124 (12.8246, 42.2853) -> (18.478, 42.2853) construction
  line L125 (18.478, 42.2853) -> (18.478, 52.8686) construction
  line L126 (18.478, 52.8686) -> (12.8246, 52.8686) construction
  line L127 (12.8246, 52.8686) -> (12.8246, 42.2853) construction
  line L128 (29.4933, 42.2853) -> (36.1699, 42.2853) construction
  line L129 (36.1699, 42.2853) -> (36.1699, 52.8686) construction
  line L130 (36.1699, 52.8686) -> (29.4933, 52.8686) construction
  line L131 (29.4933, 52.8686) -> (29.4933, 42.2853) construction
  line L132 (46.1621, 42.2853) -> (52.1669, 42.2853) construction
  line L133 (52.1669, 42.2853) -> (52.1669, 52.8686) construction
  line L134 (52.1669, 52.8686) -> (46.1621, 52.8686) construction
  line L135 (46.1621, 52.8686) -> (46.1621, 42.2853) construction
  line L136 (62.8308, 42.2853) -> (68.4842, 42.2853) construction
  line L137 (68.4842, 42.2853) -> (68.4842, 52.8686) construction
  line L138 (68.4842, 52.8686) -> (62.8308, 52.8686) construction
  line L139 (62.8308, 52.8686) -> (62.8308, 42.2853) construction
  line L140 (79.4996, 42.2853) -> (84.2331, 42.2853) construction
  line L141 (84.2331, 42.2853) -> (84.2331, 52.8686) construction
  line L142 (84.2331, 52.8686) -> (79.4996, 52.8686) construction
  line L143 (79.4996, 52.8686) -> (79.4996, 42.2853) construction
  line L144 (96.1683, 42.2853) -> (102.5183, 42.2853) construction
  line L145 (102.5183, 42.2853) -> (102.5183, 52.8686) construction
  line L146 (102.5183, 52.8686) -> (96.1683, 52.8686) construction
  line L147 (96.1683, 52.8686) -> (96.1683, 42.2853) construction
  line L148 (-87.1879, 23.7853) -> (-81.2193, 23.7853) construction
  line L149 (-81.2193, 23.7853) -> (-81.2193, 34.3686) construction
  line L150 (-81.2193, 34.3686) -> (-87.1879, 34.3686) construction
  line L151 (-87.1879, 34.3686) -> (-87.1879, 23.7853) construction
  line L152 (-70.5192, 23.7853) -> (-63.4292, 23.7853) construction
  line L153 (-63.4292, 23.7853) -> (-63.4292, 34.3686) construction
  line L154 (-63.4292, 34.3686) -> (-70.5192, 34.3686) construction
  line L155 (-70.5192, 34.3686) -> (-70.5192, 23.7853) construction
  line L156 (-53.8504, 23.7853) -> (-47.1532, 23.7853) construction
  line L157 (-47.1532, 23.7853) -> (-47.1532, 34.3686) construction
  line L158 (-47.1532, 34.3686) -> (-53.8504, 34.3686) construction
  line L159 (-53.8504, 34.3686) -> (-53.8504, 23.7853) construction
  line L160 (-37.1817, 23.7853) -> (-31.2389, 23.7853) construction
  line L161 (-31.2389, 23.7853) -> (-31.2389, 34.3686) construction
  line L162 (-31.2389, 34.3686) -> (-37.1817, 34.3686) construction
  line L163 (-37.1817, 34.3686) -> (-37.1817, 23.7853) construction
  line L164 (-20.5129, 23.7853) -> (-13.4229, 23.7853) construction
  line L165 (-13.4229, 23.7853) -> (-13.4229, 34.3686) construction
  line L166 (-13.4229, 34.3686) -> (-20.5129, 34.3686) construction
  line L167 (-20.5129, 34.3686) -> (-20.5129, 23.7853) construction
  line L168 (-3.8442, 23.7853) -> (1.9384, 23.7853) construction
  line L169 (1.9384, 23.7853) -> (1.9384, 34.3686) construction
  line L170 (1.9384, 34.3686) -> (-3.8442, 34.3686) construction
  line L171 (-3.8442, 34.3686) -> (-3.8442, 23.7853) construction
  line L172 (12.8246, 23.7853) -> (18.6072, 23.7853) construction
  line L173 (18.6072, 23.7853) -> (18.6072, 34.3686) construction
  line L174 (18.6072, 34.3686) -> (12.8246, 34.3686) construction
  line L175 (12.8246, 34.3686) -> (12.8246, 23.7853) construction
  line L176 (29.4933, 23.7853) -> (36.4386, 23.7853) construction
  line L177 (36.4386, 23.7853) -> (36.4386, 34.3686) construction
  line L178 (36.4386, 34.3686) -> (29.4933, 34.3686) construction
  line L179 (29.4933, 34.3686) -> (29.4933, 23.7853) construction
  line L180 (46.1621, 23.7853) -> (53.0919, 23.7853) construction
  line L181 (53.0919, 23.7853) -> (53.0919, 34.3686) construction
  line L182 (53.0919, 34.3686) -> (46.1621, 34.3686) construction
  line L183 (46.1621, 34.3686) -> (46.1621, 23.7853) construction
  line L184 (62.8308, 23.7853) -> (70.0759, 23.7853) construction
  line L185 (70.0759, 23.7853) -> (70.0759, 34.3686) construction
  line L186 (70.0759, 34.3686) -> (62.8308, 34.3686) construction
  line L187 (62.8308, 34.3686) -> (62.8308, 23.7853) construction
  line L188 (79.4996, 23.7853) -> (86.1762, 23.7853) construction
  line L189 (86.1762, 23.7853) -> (86.1762, 34.3686) construction
  line L190 (86.1762, 34.3686) -> (79.4996, 34.3686) construction
  line L191 (79.4996, 34.3686) -> (79.4996, 23.7853) construction
  line L192 (96.1683, 23.7853) -> (102.5183, 23.7853) construction
  line L193 (102.5183, 23.7853) -> (102.5183, 34.3686) construction
  line L194 (102.5183, 34.3686) -> (96.1683, 34.3686) construction
  line L195 (96.1683, 34.3686) -> (96.1683, 23.7853) construction
  line L196 (-87.1879, 5.2853) -> (-81.2451, 5.2853) construction
  line L197 (-81.2451, 5.2853) -> (-81.2451, 15.8686) construction
  line L198 (-81.2451, 15.8686) -> (-87.1879, 15.8686) construction
  line L199 (-87.1879, 15.8686) -> (-87.1879, 5.2853) construction
  line L200 (-70.5192, 5.2853) -> (-63.4292, 5.2853) construction
  line L201 (-63.4292, 5.2853) -> (-63.4292, 15.8686) construction
  line L202 (-63.4292, 15.8686) -> (-70.5192, 15.8686) construction
  line L203 (-70.5192, 15.8686) -> (-70.5192, 5.2853) construction
  line L204 (-53.8504, 5.2853) -> (-49.1169, 5.2853) construction
  line L205 (-49.1169, 5.2853) -> (-49.1169, 15.8686) construction
  line L206 (-49.1169, 15.8686) -> (-53.8504, 15.8686) construction
  line L207 (-53.8504, 15.8686) -> (-53.8504, 5.2853) construction
  line L208 (-37.1817, 5.2853) -> (-31.4611, 5.2853) construction
  line L209 (-31.4611, 5.2853) -> (-31.4611, 15.8686) construction
  line L210 (-31.4611, 15.8686) -> (-37.1817, 15.8686) construction
  line L211 (-37.1817, 15.8686) -> (-37.1817, 5.2853) construction
  line L212 (-17.0129, 5.2853) -> (-16.0104, 5.2853) construction
  line L213 (-16.0104, 5.2853) -> (-16.0104, 15.8686) construction
  line L214 (-16.0104, 15.8686) -> (-17.0129, 15.8686) construction
  line L215 (-17.0129, 15.8686) -> (-17.0129, 5.2853) construction
  line L216 (-3.8442, 5.2853) -> (2.8324, 5.2853) construction
  line L217 (2.8324, 5.2853) -> (2.8324, 15.8686) construction
  line L218 (2.8324, 15.8686) -> (-3.8442, 15.8686) construction
  line L219 (-3.8442, 15.8686) -> (-3.8442, 5.2853) construction
  line L220 (12.8246, 5.2853) -> (18.8294, 5.2853) construction
  line L221 (18.8294, 5.2853) -> (18.8294, 15.8686) construction
  line L222 (18.8294, 15.8686) -> (12.8246, 15.8686) construction
  line L223 (12.8246, 15.8686) -> (12.8246, 5.2853) construction
  line L224 (29.4933, 5.2853) -> (35.4361, 5.2853) construction
  line L225 (35.4361, 5.2853) -> (35.4361, 15.8686) construction
  line L226 (35.4361, 15.8686) -> (29.4933, 15.8686) construction
  line L227 (29.4933, 15.8686) -> (29.4933, 5.2853) construction
  line L228 (46.1621, 5.2853) -> (52.4253, 5.2853) construction
  line L229 (52.4253, 5.2853) -> (52.4253, 15.8686) construction
  line L230 (52.4253, 15.8686) -> (46.1621, 15.8686) construction
  line L231 (46.1621, 15.8686) -> (46.1621, 5.2853) construction
  line L232 (62.8308, 5.2853) -> (69.9208, 5.2853) construction
  line L233 (69.9208, 5.2853) -> (69.9208, 15.8686) construction
  line L234 (69.9208, 15.8686) -> (62.8308, 15.8686) construction
  line L235 (62.8308, 15.8686) -> (62.8308, 5.2853) construction
  line L236 (79.4996, 5.2853) -> (86.4449, 5.2853) construction
  line L237 (86.4449, 5.2853) -> (86.4449, 15.8686) construction
  line L238 (86.4449, 15.8686) -> (79.4996, 15.8686) construction
  line L239 (79.4996, 15.8686) -> (79.4996, 5.2853) construction
  line L240 (96.1683, 5.2853) -> (102.5183, 5.2853) construction
  line L241 (102.5183, 5.2853) -> (102.5183, 15.8686) construction
  line L242 (102.5183, 15.8686) -> (96.1683, 15.8686) construction
  line L243 (96.1683, 15.8686) -> (96.1683, 5.2853) construction
  line L244 (-87.1879, -13.2147) -> (-80.9247, -13.2147) construction
  line L245 (-80.9247, -13.2147) -> (-80.9247, -2.6314) construction
  line L246 (-80.9247, -2.6314) -> (-87.1879, -2.6314) construction
  line L247 (-87.1879, -2.6314) -> (-87.1879, -13.2147) construction
  line L248 (-70.5192, -13.2147) -> (-63.8426, -13.2147) construction
  line L249 (-63.8426, -13.2147) -> (-63.8426, -2.6314) construction
  line L250 (-63.8426, -2.6314) -> (-70.5192, -2.6314) construction
  line L251 (-70.5192, -2.6314) -> (-70.5192, -13.2147) construction
  line L252 (-53.8504, -13.2147) -> (-47.8611, -13.2147) construction
  line L253 (-47.8611, -13.2147) -> (-47.8611, -2.6314) construction
  line L254 (-47.8611, -2.6314) -> (-53.8504, -2.6314) construction
  line L255 (-53.8504, -2.6314) -> (-53.8504, -13.2147) construction
  line L256 (-37.1817, -13.2147) -> (-27.4407, -13.2147) construction
  line L257 (-27.4407, -13.2147) -> (-27.4407, -2.6314) construction
  line L258 (-27.4407, -2.6314) -> (-37.1817, -2.6314) construction
  line L259 (-37.1817, -2.6314) -> (-37.1817, -13.2147) construction
  line L260 (-20.5129, -13.2147) -> (-13.2679, -13.2147) construction
  line L261 (-13.2679, -13.2147) -> (-13.2679, -2.6314) construction
  line L262 (-13.2679, -2.6314) -> (-20.5129, -2.6314) construction
  line L263 (-20.5129, -2.6314) -> (-20.5129, -13.2147) construction
  line L264 (-3.8442, -13.2147) -> (0.8894, -13.2147) construction
  line L265 (0.8894, -13.2147) -> (0.8894, -2.6314) construction
  line L266 (0.8894, -2.6314) -> (-3.8442, -2.6314) construction
  line L267 (-3.8442, -2.6314) -> (-3.8442, -13.2147) construction
  line L268 (12.8246, -13.2147) -> (17.9354, -13.2147) construction
  line L269 (17.9354, -13.2147) -> (17.9354, -2.6314) construction
  line L270 (17.9354, -2.6314) -> (12.8246, -2.6314) construction
  line L271 (12.8246, -2.6314) -> (12.8246, -13.2147) construction
  line L272 (29.4933, -13.2147) -> (35.4516, -13.2147) construction
  line L273 (35.4516, -13.2147) -> (35.4516, -2.6314) construction
  line L274 (35.4516, -2.6314) -> (29.4933, -2.6314) construction
  line L275 (29.4933, -2.6314) -> (29.4933, -13.2147) construction
  line L276 (46.1621, -13.2147) -> (52.1307, -13.2147) construction
  line L277 (52.1307, -13.2147) -> (52.1307, -2.6314) construction
  line L278 (52.1307, -2.6314) -> (46.1621, -2.6314) construction
  line L279 (46.1621, -2.6314) -> (46.1621, -13.2147) construction
  line L280 (62.8308, -13.2147) -> (67.9416, -13.2147) construction
  line L281 (67.9416, -13.2147) -> (67.9416, -2.6314) construction
  line L282 (67.9416, -2.6314) -> (62.8308, -2.6314) construction
  line L283 (62.8308, -2.6314) -> (62.8308, -13.2147) construction
  line L284 (79.4996, -13.2147) -> (86.4449, -13.2147) construction
  line L285 (86.4449, -13.2147) -> (86.4449, -2.6314) construction
  line L286 (86.4449, -2.6314) -> (79.4996, -2.6314) construction
  line L287 (79.4996, -2.6314) -> (79.4996, -13.2147) construction
  line L288 (96.1683, -13.2147) -> (102.5183, -13.2147) construction
  line L289 (102.5183, -13.2147) -> (102.5183, -2.6314) construction
  line L290 (102.5183, -2.6314) -> (96.1683, -2.6314) construction
  line L291 (96.1683, -2.6314) -> (96.1683, -13.2147) construction
  line L292 (-87.1879, -31.7147) -> (-81.1986, -31.7147) construction
  line L293 (-81.1986, -31.7147) -> (-81.1986, -21.1314) construction
  line L294 (-81.1986, -21.1314) -> (-87.1879, -21.1314) construction
  line L295 (-87.1879, -21.1314) -> (-87.1879, -31.7147) construction
  line L296 (-70.5192, -31.7147) -> (-64.8658, -31.7147) construction
  line L297 (-64.8658, -31.7147) -> (-64.8658, -21.1314) construction
  line L298 (-64.8658, -21.1314) -> (-70.5192, -21.1314) construction
  line L299 (-70.5192, -21.1314) -> (-70.5192, -31.7147) construction
  line L300 (-53.8504, -31.7147) -> (-47.9076, -31.7147) construction
  line L301 (-47.9076, -31.7147) -> (-47.9076, -21.1314) construction
  line L302 (-47.9076, -21.1314) -> (-53.8504, -21.1314) construction
  line L303 (-53.8504, -21.1314) -> (-53.8504, -31.7147) construction
  line L304 (-37.1817, -31.7147) -> (-31.213, -31.7147) construction
  line L305 (-31.213, -31.7147) -> (-31.213, -21.1314) construction
  line L306 (-31.213, -21.1314) -> (-37.1817, -21.1314) construction
  line L307 (-37.1817, -21.1314) -> (-37.1817, -31.7147) construction
  line L308 (-20.5129, -31.7147) -> (-14.8595, -31.7147) construction
  line L309 (-14.8595, -31.7147) -> (-14.8595, -21.1314) construction
  line L310 (-14.8595, -21.1314) -> (-20.5129, -21.1314) construction
  line L311 (-20.5129, -21.1314) -> (-20.5129, -31.7147) construction
  line L312 (-3.8442, -31.7147) -> (2.1141, -31.7147) construction
  line L313 (2.1141, -31.7147) -> (2.1141, -21.1314) construction
  line L314 (2.1141, -21.1314) -> (-3.8442, -21.1314) construction
  line L315 (-3.8442, -21.1314) -> (-3.8442, -31.7147) construction
  line L316 (12.8246, -31.7147) -> (18.7932, -31.7147) construction
  line L317 (18.7932, -31.7147) -> (18.7932, -21.1314) construction
  line L318 (18.7932, -21.1314) -> (12.8246, -21.1314) construction
  line L319 (12.8246, -21.1314) -> (12.8246, -31.7147) construction
  line L320 (29.4933, -31.7147) -> (35.7565, -31.7147) construction
  line L321 (35.7565, -31.7147) -> (35.7565, -21.1314) construction
  line L322 (35.7565, -21.1314) -> (29.4933, -21.1314) construction
  line L323 (29.4933, -21.1314) -> (29.4933, -31.7147) construction
  line L324 (46.1621, -31.7147) -> (52.8387, -31.7147) construction
  line L325 (52.8387, -31.7147) -> (52.8387, -21.1314) construction
  line L326 (52.8387, -21.1314) -> (46.1621, -21.1314) construction
  line L327 (46.1621, -21.1314) -> (46.1621, -31.7147) construction
  line L328 (62.8308, -31.7147) -> (68.4842, -31.7147) construction
  line L329 (68.4842, -31.7147) -> (68.4842, -21.1314) construction
  line L330 (68.4842, -21.1314) -> (62.8308, -21.1314) construction
  line L331 (62.8308, -21.1314) -> (62.8308, -31.7147) construction
  line L332 (82.9996, -31.7147) -> (84.0021, -31.7147) construction
  line L333 (84.0021, -31.7147) -> (84.0021, -21.1314) construction
  line L334 (84.0021, -21.1314) -> (82.9996, -21.1314) construction
  line L335 (82.9996, -21.1314) -> (82.9996, -31.7147) construction
  line L336 (96.1683, -31.7147) -> (102.5183, -31.7147) construction
  line L337 (102.5183, -31.7147) -> (102.5183, -21.1314) construction
  line L338 (102.5183, -21.1314) -> (96.1683, -21.1314) construction
  line L339 (96.1683, -21.1314) -> (96.1683, -31.7147) construction
  line L340 (-87.1879, -50.2147) -> (-81.1986, -50.2147) construction
  line L341 (-81.1986, -50.2147) -> (-81.1986, -39.6314) construction
  line L342 (-81.1986, -39.6314) -> (-87.1879, -39.6314) construction
  line L343 (-87.1879, -39.6314) -> (-87.1879, -50.2147) construction
  line L344 (-70.5192, -50.2147) -> (-60.7782, -50.2147) construction
  line L345 (-60.7782, -50.2147) -> (-60.7782, -39.6314) construction
  line L346 (-60.7782, -39.6314) -> (-70.5192, -39.6314) construction
  line L347 (-70.5192, -39.6314) -> (-70.5192, -50.2147) construction
  line L348 (-53.8504, -50.2147) -> (-48.197, -50.2147) construction
  line L349 (-48.197, -50.2147) -> (-48.197, -39.6314) construction
  line L350 (-48.197, -39.6314) -> (-53.8504, -39.6314) construction
  line L351 (-53.8504, -39.6314) -> (-53.8504, -50.2147) construction
  line L352 (-33.6817, -50.2147) -> (-32.6791, -50.2147) construction
  line L353 (-32.6791, -50.2147) -> (-32.6791, -39.6314) construction
  line L354 (-32.6791, -39.6314) -> (-33.6817, -39.6314) construction
  line L355 (-33.6817, -39.6314) -> (-33.6817, -50.2147) construction
  line L356 (-20.5129, -50.2147) -> (-14.5443, -50.2147) construction
  line L357 (-14.5443, -50.2147) -> (-14.5443, -39.6314) construction
  line L358 (-14.5443, -39.6314) -> (-20.5129, -39.6314) construction
  line L359 (-20.5129, -39.6314) -> (-20.5129, -50.2147) construction
  line L360 (-3.8442, -50.2147) -> (2.1865, -50.2147) construction
  line L361 (2.1865, -50.2147) -> (2.1865, -39.6314) construction
  line L362 (2.1865, -39.6314) -> (-3.8442, -39.6314) construction
  line L363 (-3.8442, -39.6314) -> (-3.8442, -50.2147) construction
  line L364 (16.3246, -50.2147) -> (17.3271, -50.2147) construction
  line L365 (17.3271, -50.2147) -> (17.3271, -39.6314) construction
  line L366 (17.3271, -39.6314) -> (16.3246, -39.6314) construction
  line L367 (16.3246, -39.6314) -> (16.3246, -50.2147) construction
  line L368 (29.4933, -50.2147) -> (35.1467, -50.2147) construction
  line L369 (35.1467, -50.2147) -> (35.1467, -39.6314) construction
  line L370 (35.1467, -39.6314) -> (29.4933, -39.6314) construction
  line L371 (29.4933, -39.6314) -> (29.4933, -50.2147) construction
  line L372 (46.1621, -50.2147) -> (51.8827, -50.2147) construction
  line L373 (51.8827, -50.2147) -> (51.8827, -39.6314) construction
  line L374 (51.8827, -39.6314) -> (46.1621, -39.6314) construction
  line L375 (46.1621, -39.6314) -> (46.1621, -50.2147) construction
  line L376 (62.8308, -50.2147) -> (68.4842, -50.2147) construction
  line L377 (68.4842, -50.2147) -> (68.4842, -39.6314) construction
  line L378 (68.4842, -39.6314) -> (62.8308, -39.6314) construction
  line L379 (62.8308, -39.6314) -> (62.8308, -50.2147) construction
  line L380 (79.4996, -50.2147) -> (85.4682, -50.2147) construction
  line L381 (85.4682, -50.2147) -> (85.4682, -39.6314) construction
  line L382 (85.4682, -39.6314) -> (79.4996, -39.6314) construction
  line L383 (79.4996, -39.6314) -> (79.4996, -50.2147) construction
  line L384 (96.1683, -50.2147) -> (102.5183, -50.2147) construction
  line L385 (102.5183, -50.2147) -> (102.5183, -39.6314) construction
  line L386 (102.5183, -39.6314) -> (96.1683, -39.6314) construction
  line L387 (96.1683, -39.6314) -> (96.1683, -50.2147) construction